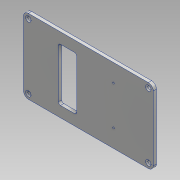
# Autodesk Inventor part: AK-C-C39-Top
Saved by Autodesk Inventor 2016 (Build 200138000, 138)
## iProperties
Created: 2016-04-01
Part Number: AK-C-C39-Top
Material: Aluminum 6061
Document SubType Name: Modeling
Designer: admin
Density: 2.7 g/cm^3
Appearance: Aluminum - Flat
Mass: 59.7394 g
Surface Area: 163.872 cm^2
Volume: 22.1257 cm^3
Author: admin
Autodesk Inventor part; units mm, degrees
ref_plane "YZ Plane" through (0, 0, 0) normal (1, 0, 0) x (0, 1, 0)
ref_plane "XZ Plane" through (0, 0, 0) normal (0, 1, 0) x (-1, 0, 0)
ref_plane "XY Plane" through (0, 0, 0) normal (0, 0, 1) x (1, 0, 0)
derived "AK-C-C39-Main-Board.ipt"
sketch "Sketch1" plane through (0, 0, 0) normal (0, 1, 0) x (-1, 0, 0)
  line L0 (-55, -17.425) -> (-56.5, -17.425)
  line L1 (-56.5, -17.425) -> (-56.5, -16.775)
  line L2 (-58.5, -16.775) -> (-58.5, -17.425)
  line L3 (-58.5, -17.425) -> (-60, -17.425)
  line L4 (-60, -29.925) -> (-60, -17.425)
  line L5 (-60, -16.775) -> (-60, 29.925)
  line L6 (55, -17.425) -> (56.5, -17.425)
  line L7 (58.5, -17.425) -> (60, -17.425)
  line L8 (60, -29.925) -> (60, -17.425)
  line L9 (60, -16.775) -> (60, 29.925)
  arc A0 (-52.8, -29.7756) -> (-53.6536, -29.4221) centre (-53.3, -29.7756) ccw
  arc A1 (-54.9971, -28.0786) -> (-55.3506, -27.225) centre (-55.3506, -27.725) ccw
  line L10 (-54.2538, -30.0223) -> (-53.6536, -29.4221)
  line L11 (-55.5973, -28.6788) -> (-54.9971, -28.0786)
  arc A2 (54.9971, 28.0786) -> (55.3506, 27.225) centre (55.3506, 27.725) ccw
  line L12 (55.5, 29.925) -> (51.9091, 26.3341) construction
  arc A3 (52.8, 29.7756) -> (53.6536, 29.4221) centre (53.3, 29.7756) ccw
  line L13 (55, -16.775) -> (56.5, -16.775)
  line L14 (58.5, -16.775) -> (60, -16.775)
  line L15 (57.8, -3.3607) -> (55, -7.6074)
  line L16 (55, -7.6074) -> (55, -16.775)
  arc A4 (56.5, -18.525) -> (58.5, -18.525) centre (57.5, -19.275) ccw
  line L17 (58.5, -18.525) -> (58.5, -16.775)
  line L18 (56.5, -18.525) -> (56.5, -16.775)
  line L19 (-55.5973, 28.6788) -> (-54.9971, 28.0786)
  line L20 (-54.2538, 30.0223) -> (-53.6536, 29.4221)
  arc A5 (-53.6536, 29.4221) -> (-52.8, 29.7756) centre (-53.3, 29.7756) ccw
  arc A6 (-55.3506, 27.225) -> (-54.9971, 28.0786) centre (-55.3506, 27.725) ccw
  line L21 (-57.8, -3.3607) -> (-55, -7.6074)
  line L22 (-55, -7.6074) -> (-55, -16.775)
  arc A7 (-56.5, -15.025) -> (-58.5, -15.025) centre (-57.5, -14.275) ccw
  line L23 (-58.5, -15.025) -> (-58.5, -16.775)
  line L24 (-56.5, -15.025) -> (-56.5, -16.775)
  line L25 (-55, -16.775) -> (-56.5, -16.775)
  line L26 (-58.5, -16.775) -> (-60, -16.775)
  line L27 (57.5, -16.4962) -> (57.5, -11.7384) construction
  line L28 (-52.8, -31.925) -> (-52.8, -29.7756)
  line L29 (-55.3506, -27.225) -> (-57.5, -27.225)
  line L30 (-57.5, -27.225) -> (-57.5, -25.225)
  line L31 (-57.5, -25.225) -> (-55, -25.225)
  line L32 (-55, -25.225) -> (-55, -17.425)
  line L33 (48.8, -31.925) -> (46.8, -31.925)
  line L34 (46.8, -31.925) -> (46.8, -29.925)
  line L35 (46.8, -29.925) -> (44.8, -29.925)
  line L36 (44.8, -29.925) -> (44.8, -32.325)
  line L37 (-44.8, -32.325) -> (-44.8, -29.925)
  line L38 (-44.8, -29.925) -> (-46.8, -29.925)
  line L39 (-46.8, -29.925) -> (-46.8, -31.925)
  line L40 (-46.8, -31.925) -> (-48.8, -31.925)
  line L41 (-48.8, -31.925) -> (-48.8, -29.925)
  line L42 (-48.8, -29.925) -> (-50.8, -29.925)
  line L43 (-50.8, -29.925) -> (-50.8, -31.925)
  line L44 (-50.8, -31.925) -> (-52.8, -31.925)
  line L45 (55, -17.425) -> (55, -25.225)
  line L46 (55, -25.225) -> (57.5, -25.225)
  line L47 (57.5, -25.225) -> (57.5, -27.225)
  line L48 (57.5, -27.225) -> (55.3506, -27.225)
  line L49 (52.8, -29.7756) -> (52.8, -31.925)
  line L50 (52.8, -31.925) -> (50.8, -31.925)
  line L51 (50.8, -31.925) -> (50.8, -29.925)
  line L52 (50.8, -29.925) -> (48.8, -29.925)
  line L53 (48.8, -29.925) -> (48.8, -31.925)
  line L54 (5, -32.325) -> (5, -29.925)
  line L55 (5, -29.925) -> (3, -29.925)
  line L56 (3, -29.925) -> (3, -31.925)
  line L57 (3, -31.925) -> (1, -31.925)
  line L58 (1, -31.925) -> (1, -29.925)
  line L59 (1, -29.925) -> (-1, -29.925)
  line L60 (-1, -29.925) -> (-1, -31.925)
  line L61 (-1, -31.925) -> (-3, -31.925)
  line L62 (-3, -31.925) -> (-3, -29.925)
  line L63 (-3, -29.925) -> (-5, -29.925)
  line L64 (-5, -29.925) -> (-5, -32.325)
  line L65 (-5, -32.325) -> (-44.8, -32.325)
  line L66 (44.8, -32.325) -> (5, -32.325)
  line L67 (-57.5, -20.9142) -> (-57.5, -16.6435) construction
  arc A8 (60, 29.925) -> (55.5, 34.425) centre (55.5, 29.925) ccw
  arc A9 (-55.5, 34.425) -> (-60, 29.925) centre (-55.5, 29.925) ccw
  arc A10 (-60, -29.925) -> (-55.5, -34.425) centre (-55.5, -29.925) ccw
  line L68 (57.5, 27.225) -> (57.5, 25.225)
  line L69 (57.5, 25.225) -> (55.5, 25.225)
  line L70 (55.5, 25.225) -> (55.5, 23.225)
  line L71 (55.5, 23.225) -> (57.5, 23.225)
  line L72 (57.5, 23.225) -> (57.5, 21.225)
  line L73 (57.5, 21.225) -> (55.5, 21.225)
  line L74 (55.5, 21.225) -> (55.5, 19.225)
  line L75 (55.5, 19.225) -> (57.8, 19.225)
  line L76 (57.8, 19.225) -> (57.8, -3.3607)
  line L77 (3, 31.925) -> (1, 31.925)
  line L78 (1, 31.925) -> (1, 29.925)
  line L79 (1, 29.925) -> (-1, 29.925)
  line L80 (-1, 29.925) -> (-1, 31.925)
  line L81 (-1, 31.925) -> (-3, 31.925)
  line L82 (-3, 31.925) -> (-3, 29.925)
  line L83 (-3, 29.925) -> (-5, 29.925)
  line L84 (-5, 29.925) -> (-5, 32.325)
  line L85 (-5, 32.325) -> (-44.8, 32.325)
  line L86 (-44.8, 32.325) -> (-44.8, 29.925)
  line L87 (-44.8, 29.925) -> (-46.8, 29.925)
  line L88 (-46.8, 29.925) -> (-46.8, 31.925)
  line L89 (-46.8, 31.925) -> (-48.8, 31.925)
  line L90 (-48.8, 31.925) -> (-48.8, 29.925)
  line L91 (-48.8, 29.925) -> (-50.8, 29.925)
  line L92 (-50.8, 29.925) -> (-50.8, 31.925)
  line L93 (-50.8, 31.925) -> (-52.8, 31.925)
  line L94 (-52.8, 31.925) -> (-52.8, 29.7756)
  line L95 (-55.3506, 27.225) -> (-57.5, 27.225)
  line L96 (55.5973, 28.6788) -> (54.9971, 28.0786)
  line L97 (54.2538, 30.0223) -> (53.6536, 29.4221)
  line L98 (57.5, 27.225) -> (55.3506, 27.225)
  line L99 (52.8, 29.7756) -> (52.8, 31.925)
  line L100 (52.8, 31.925) -> (50.8, 31.925)
  line L101 (50.8, 31.925) -> (50.8, 29.925)
  line L102 (50.8, 29.925) -> (48.8, 29.925)
  line L103 (48.8, 29.925) -> (48.8, 31.925)
  line L104 (48.8, 31.925) -> (46.8, 31.925)
  line L105 (46.8, 31.925) -> (46.8, 29.925)
  line L106 (46.8, 29.925) -> (44.8, 29.925)
  line L107 (44.8, 29.925) -> (44.8, 32.325)
  line L108 (44.8, 32.325) -> (5, 32.325)
  line L109 (5, 32.325) -> (5, 29.925)
  line L110 (5, 29.925) -> (3, 29.925)
  line L111 (3, 29.925) -> (3, 31.925)
  line L112 (-57.5, 27.225) -> (-57.5, 25.225)
  line L113 (-57.5, 25.225) -> (-55.5, 25.225)
  line L114 (-55.5, 25.225) -> (-55.5, 23.225)
  line L115 (-55.5, 23.225) -> (-57.5, 23.225)
  line L116 (-57.5, 23.225) -> (-57.5, 21.225)
  line L117 (-57.5, 21.225) -> (-55.5, 21.225)
  line L118 (-55.5, 21.225) -> (-55.5, 19.225)
  line L119 (-55.5, 19.225) -> (-57.8, 19.225)
  line L120 (-57.8, 19.225) -> (-57.8, -3.3607)
  line L121 (55.5, -34.425) -> (-55.5, -34.425)
  line L122 (9.5866, 0) -> (-6.7847, 0) construction
  line L123 (0, -6.6233) -> (0, 6.4737) construction
  arc A11 (55.5, -34.425) -> (60, -29.925) centre (55.5, -29.925) ccw
  arc A12 (55.3506, -27.225) -> (54.9971, -28.0786) centre (55.3506, -27.725) ccw
  arc A13 (53.6536, -29.4221) -> (52.8, -29.7756) centre (53.3, -29.7756) ccw
  line L124 (54.9971, -28.0786) -> (55.5973, -28.6788)
  line L125 (53.6536, -29.4221) -> (54.2538, -30.0223)
  arc A14 (55.5973, 28.6788) -> (54.2538, 30.0223) centre (55.5, 29.925) ccw
  arc A15 (-54.2538, 30.0223) -> (-55.5973, 28.6788) centre (-55.5, 29.925) ccw
  arc A16 (54.2538, -30.0223) -> (55.5973, -28.6788) centre (55.5, -29.925) ccw
  arc A17 (-55.5973, -28.6788) -> (-54.2538, -30.0223) centre (-55.5, -29.925) ccw
  line L126 (55.5, 34.425) -> (-55.5, 34.425)
  point P0 (0, 0)
sketch "Sketch2" plane through (0, 0, 0) normal (0, 1, 0) x (-1, 0, 0)
  line L0 (51.25, -29) -> (44.125, -29)
  line L1 (43.25, -29.875) -> (43.25, -31)
  line L2 (43.25, -31) -> (6.5, -31)
  line L3 (6.5, -31) -> (6.5, -29.875)
  line L4 (5.625, -29) -> (-5.625, -29)
  line L5 (-6.5, -29.875) -> (-6.5, -31)
  line L6 (-6.5, -31) -> (-43.25, -31)
  line L7 (-43.25, -31) -> (-43.25, -29.875)
  line L8 (-44.125, -29) -> (-51.25, -29)
  line L9 (-51.25, -29) -> (-53.75, -26.5)
  line L10 (-53.75, -26.5) -> (-53.75, 26.5)
  line L11 (-53.75, 26.5) -> (-51.25, 29)
  line L12 (-51.25, 29) -> (-44.125, 29)
  line L13 (-43.25, 29.875) -> (-43.25, 31)
  line L14 (-43.25, 31) -> (-6.5, 31)
  line L15 (-6.5, 31) -> (-6.5, 29.875)
  line L16 (-5.625, 29) -> (5.625, 29)
  line L17 (6.5, 29.875) -> (6.5, 31)
  line L18 (43.25, 31) -> (43.25, 29.875)
  line L19 (43.25, 31) -> (6.5, 31)
  line L20 (44.125, 29) -> (51.25, 29)
  line L21 (51.25, 29) -> (53.75, 26.5)
  line L22 (53.75, 26.5) -> (53.75, -26.5)
  line L23 (53.75, -26.5) -> (51.25, -29)
  line L24 (44.8, -32.325) -> (5, -32.325)
  line L25 (5, -32.325) -> (5, -29.925)
  line L26 (5, -29.925) -> (3, -29.925)
  line L27 (44.8, -29.925) -> (44.8, -32.325)
  line L28 (46.8, -29.925) -> (44.8, -29.925)
  line L29 (52.8, -29.7756) -> (52.8, -31.925)
  arc A0 (53.6536, -29.4221) -> (52.8, -29.7756) centre (53.3, -29.7756) ccw
  arc A1 (55.3506, -27.225) -> (54.9971, -28.0786) centre (55.3506, -27.725) ccw
  line L30 (55, -17.425) -> (55, -25.225)
  line L31 (0, -6.6233) -> (0, 6.4737) construction
  line L32 (9.5866, 0) -> (-6.7847, 0) construction
  line L33 (57.8, 19.225) -> (57.8, -3.3607)
  line L34 (57.8, -3.3607) -> (55, -7.6074)
  line L35 (55.5, 19.225) -> (57.8, 19.225)
  line L36 (55.5, 29.925) -> (51.9091, 26.3341) construction
  line L37 (25.75, -24.5) -> (12.75, -24.5)
  line L38 (12.75, 24.5) -> (25.75, 24.5)
  line L39 (3.3524, -20) -> (-16.6476, -20)
  line L40 (-16.6476, -20) -> (-16.6476, 20)
  line L41 (-16.6476, 20) -> (3.3524, 20)
  line L42 (3.3524, 20) -> (3.3524, -20)
  line L43 (-23.9878, -15) -> (-31.9878, -15) construction
  line L44 (-31.9878, -15) -> (-31.9878, -7) construction
  line L45 (-31.9878, -7) -> (-23.9878, -7) construction
  line L46 (-23.9878, -7) -> (-23.9878, -15) construction
  line L47 (-34.9878, -15) -> (-42.9878, -15) construction
  line L48 (-42.9878, -15) -> (-42.9878, -7) construction
  line L49 (-42.9878, -7) -> (-34.9878, -7) construction
  line L50 (-34.9878, -7) -> (-34.9878, -15) construction
  line L51 (-23.9878, -4) -> (-31.9878, -4) construction
  line L52 (-31.9878, -4) -> (-31.9878, 4) construction
  line L53 (-31.9878, 4) -> (-23.9878, 4) construction
  line L54 (-23.9878, 4) -> (-23.9878, -4) construction
  line L55 (-34.9878, -4) -> (-42.9878, -4) construction
  line L56 (-42.9878, -4) -> (-42.9878, 4) construction
  line L57 (-42.9878, 4) -> (-34.9878, 4) construction
  line L58 (-34.9878, 4) -> (-34.9878, -4) construction
  line L59 (-23.9878, 7) -> (-31.9878, 7) construction
  line L60 (-31.9878, 7) -> (-31.9878, 15) construction
  line L61 (-31.9878, 15) -> (-23.9878, 15) construction
  line L62 (-23.9878, 15) -> (-23.9878, 7) construction
  line L63 (-34.9878, 7) -> (-42.9878, 7) construction
  line L64 (-42.9878, 7) -> (-42.9878, 15) construction
  line L65 (-42.9878, 15) -> (-34.9878, 15) construction
  line L66 (-34.9878, 15) -> (-34.9878, 7) construction
  line L67 (25.75, -22.5) -> (12.75, -22.5) construction
  line L68 (12.75, -22.5) -> (12.75, -9.5) construction
  line L69 (12.75, -9.5) -> (25.75, -9.5) construction
  line L70 (25.75, -9.5) -> (25.75, -22.5) construction
  line L71 (25.75, -6.5) -> (12.75, -6.5) construction
  line L72 (12.75, -6.5) -> (12.75, 6.5) construction
  line L73 (12.75, 6.5) -> (25.75, 6.5) construction
  line L74 (25.75, 6.5) -> (25.75, -6.5) construction
  line L75 (25.75, 9.5) -> (12.75, 9.5) construction
  line L76 (12.75, 9.5) -> (12.75, 22.5) construction
  line L77 (12.75, 22.5) -> (25.75, 22.5) construction
  line L78 (25.75, 22.5) -> (25.75, 9.5) construction
  line L79 (31.9633, -16) -> (17.7262, -16) construction
  line L80 (31.9633, 16) -> (18.8213, 16) construction
  line L81 (19.25, -23.7063) -> (19.25, 24.6931) construction
  arc A2 (10.75, -22.5) -> (12.75, -24.5) centre (12.75, -22.5) ccw
  arc A3 (25.75, -24.5) -> (27.75, -22.5) centre (25.75, -22.5) ccw
  arc A4 (12.75, 24.5) -> (10.75, 22.5) centre (12.75, 22.5) ccw
  arc A5 (27.75, 22.5) -> (25.75, 24.5) centre (25.75, 22.5) ccw
  line L82 (55, -25.225) -> (-54.9956, -25.225) construction
  line L83 (55.5, 25.225) -> (55.5, 23.225)
  line L84 (57.5, 25.225) -> (55.5, 25.225)
  line L85 (-57.5, 25.225) -> (-55.5, 25.225)
  line L86 (-55.5, 25.225) -> (-55.5, 23.225)
  line L87 (-57.5, -25.225) -> (-55, -25.225)
  line L88 (-55, -25.225) -> (-55, -17.425)
  line L89 (55, -25.225) -> (57.5, -25.225)
  line L90 (55.5, 25.225) -> (-55.5, 25.225) construction
  line L91 (48.25, -2.5) -> (48.25, 2.5)
  line L92 (50, -2.5) -> (50, 2.5)
  line L93 (50, -4) -> (48.25, -4)
  line L94 (50, 4) -> (48.25, 4)
  arc A6 (50, -4) -> (50, -2.5) centre (50, -3.25) ccw
  arc A7 (48.25, -2.5) -> (48.25, -4) centre (48.25, -3.25) ccw
  arc A8 (50, 2.5) -> (50, 4) centre (50, 3.25) ccw
  arc A9 (48.25, 4) -> (48.25, 2.5) centre (48.25, 3.25) ccw
  line L95 (-37.75, -2.5) -> (-37.75, 2.5)
  line L96 (-39.5, 4) -> (-37.75, 4)
  line L97 (-39.5, 2.5) -> (-39.5, -2.5)
  line L98 (-39.5, -4) -> (-37.75, -4)
  arc A10 (-37.75, -4) -> (-37.75, -2.5) centre (-37.75, -3.25) ccw
  arc A11 (-39.5, -2.5) -> (-39.5, -4) centre (-39.5, -3.25) ccw
  arc A12 (-37.75, 2.5) -> (-37.75, 4) centre (-37.75, 3.25) ccw
  arc A13 (-39.5, 4) -> (-39.5, 2.5) centre (-39.5, 3.25) ccw
  line L99 (48.75, -27) -> (40.5, -27)
  line L100 (38.75, -27) -> (38.75, -25.25)
  line L101 (40.5, -25.25) -> (48.75, -25.25)
  line L102 (1.75, -27) -> (-8.25, -27)
  line L103 (-8.25, -25.25) -> (1.75, -25.25)
  line L104 (-40, -27) -> (-48.25, -27)
  line L105 (-48.25, -25.25) -> (-40, -25.25)
  line L106 (-48.25, 25.25) -> (-40, 25.25)
  line L107 (-40, 27) -> (-48.25, 27)
  line L108 (1.75, 25.25) -> (-8.25, 25.25)
  line L109 (-8.25, 27) -> (1.75, 27)
  line L110 (48.75, 25.25) -> (40.25, 25.25)
  line L111 (38.75, 25.25) -> (38.75, 27)
  line L112 (40.25, 27) -> (48.75, 27)
  arc A14 (38.75, -27) -> (40.5, -27) centre (39.625, -27) ccw
  arc A15 (40.5, -25.25) -> (38.75, -25.25) centre (39.625, -25.25) ccw
  arc A16 (38.75, 25.25) -> (40.25, 25.25) centre (39.5, 25.25) ccw
  arc A17 (40.25, 27) -> (38.75, 27) centre (39.5, 27) ccw
  line L113 (27.75, 22.5) -> (27.75, -22.5)
  line L114 (-34.9878, 7) -> (-42.9878, 15) construction
  line L115 (-31.9878, 7) -> (-23.9878, 15) construction
  line L116 (-31.9878, -7) -> (-23.9878, -15) construction
  line L117 (-34.9878, -7) -> (-42.9878, -15) construction
  arc A18 (3.3524, 19) -> (2.3524, 20) centre (2.3524, 19) ccw
  arc A19 (-15.6476, 20) -> (-16.6476, 19) centre (-15.6476, 19) ccw
  arc A20 (2.3524, -20) -> (3.3524, -19) centre (2.3524, -19) ccw
  arc A21 (-16.6476, -19) -> (-15.6476, -20) centre (-15.6476, -19) ccw
  line L118 (10.75, 7.999) -> (10.75, 8)
  line L119 (10.75, -22.5) -> (10.75, 22.5)
  arc A22 (48.75, 25.25) -> (48.75, 27) centre (48.75, 26.125) ccw
  arc A23 (-8.25, 27) -> (-8.25, 25.25) centre (-8.25, 26.125) ccw
  arc A24 (-48.25, 27) -> (-48.25, 25.25) centre (-48.25, 26.125) ccw
  arc A25 (48.75, -27) -> (48.75, -25.25) centre (48.75, -26.125) ccw
  arc A26 (-8.25, -25.25) -> (-8.25, -27) centre (-8.25, -26.125) ccw
  arc A27 (-48.25, -25.25) -> (-48.25, -27) centre (-48.25, -26.125) ccw
  line L120 (31, 25) -> (29.25, 25)
  line L121 (31, 23.5) -> (31, 20)
  line L122 (29.25, 20) -> (29.25, 23.5)
  arc A28 (31, 23.5) -> (31, 25) centre (31, 24.25) ccw
  arc A29 (29.25, 25) -> (29.25, 23.5) centre (29.25, 24.25) ccw
  arc A30 (29.25, 20) -> (31, 20) centre (30.125, 20) ccw
  line L123 (29.25, -20) -> (29.25, -23.25)
  line L124 (29.25, -25) -> (31, -25)
  line L125 (31, -23.25) -> (31, -20)
  arc A31 (31, -25) -> (31, -23.25) centre (31, -24.125) ccw
  arc A32 (29.25, -23.25) -> (29.25, -25) centre (29.25, -24.125) ccw
  arc A33 (31, -20) -> (29.25, -20) centre (30.125, -20) ccw
  line L126 (9.25, 25) -> (7.5, 25)
  line L127 (7.5, 23.5) -> (7.5, 20)
  line L128 (9.25, 20) -> (9.25, 23.5)
  line L129 (7.5, -20) -> (7.5, -23.25)
  line L130 (7.5, -25) -> (9.25, -25)
  line L131 (9.25, -23.25) -> (9.25, -20)
  arc A34 (9.25, -20) -> (7.5, -20) centre (8.375, -20) ccw
  arc A35 (9.25, -25) -> (9.25, -23.25) centre (9.25, -24.125) ccw
  arc A36 (7.5, -23.25) -> (7.5, -25) centre (7.5, -24.125) ccw
  arc A37 (7.5, 20) -> (9.25, 20) centre (8.375, 20) ccw
  arc A38 (9.25, 23.5) -> (9.25, 25) centre (9.25, 24.25) ccw
  arc A39 (7.5, 25) -> (7.5, 23.5) centre (7.5, 24.25) ccw
  line L132 (29.25, 4) -> (29.25, -4)
  line L133 (31, -4) -> (31, 4)
  line L134 (7.5, 4) -> (7.5, -4)
  line L135 (9.25, -4) -> (9.25, 4)
  arc A40 (31, 4) -> (29.25, 4) centre (30.125, 4) ccw
  arc A41 (29.25, -4) -> (31, -4) centre (30.125, -4) ccw
  arc A42 (9.25, 4) -> (7.5, 4) centre (8.375, 4) ccw
  arc A43 (7.5, -4) -> (9.25, -4) centre (8.375, -4) ccw
  line L136 (-14.75, 30.3253) -> (-31.75, 30.3253) construction
  line L137 (-31.75, 30.3253) -> (-31.75, 22.4164) construction
  line L138 (-31.75, 22.4164) -> (-14.75, 22.4164) construction
  line L139 (-14.75, 22.4164) -> (-14.75, 30.3253) construction
  line L140 (-23.25, 29.9722) -> (-23.25, 20.9797) construction
  arc A44 (6.5, -29.875) -> (5.625, -29) centre (5.625, -29.875) ccw
  arc A45 (-5.625, -29) -> (-6.5, -29.875) centre (-5.625, -29.875) ccw
  arc A46 (-43.25, -29.875) -> (-44.125, -29) centre (-44.125, -29.875) ccw
  arc A47 (-44.125, 29) -> (-43.25, 29.875) centre (-44.125, 29.875) ccw
  arc A48 (-6.5, 29.875) -> (-5.625, 29) centre (-5.625, 29.875) ccw
  arc A49 (5.625, 29) -> (6.5, 29.875) centre (5.625, 29.875) ccw
  arc A50 (43.25, 29.875) -> (44.125, 29) centre (44.125, 29.875) ccw
  arc A51 (44.125, -29) -> (43.25, -29.875) centre (44.125, -29.875) ccw
  line L141 (57.5, 27.225) -> (57.5, 25.225)
  line L142 (-57.5, 27.225) -> (-57.5, 25.225)
  arc A52 (1.75, 25.25) -> (1.75, 27) centre (1.75, 26.125) ccw
  arc A53 (1.75, -27) -> (1.75, -25.25) centre (1.75, -26.125) ccw
  arc A54 (-38.25, 27) -> (-40, 27) centre (-39.125, 27) ccw
  arc A55 (-40, 25.25) -> (-38.25, 25.25) centre (-39.125, 25.25) ccw
  line L143 (-38.25, 27) -> (-38.25, 25.25)
  arc A56 (-38.25, -25.25) -> (-40, -25.25) centre (-39.125, -25.25) ccw
  arc A57 (-40, -27) -> (-38.25, -27) centre (-39.125, -27) ccw
  line L144 (-38.25, -25.25) -> (-38.25, -27)
  line L145 (-60, -16.775) -> (-60, 29.925)
  point P0 (53.75, -25.225)
  point P1 (25.75, -16)
  point P2 (25.75, 16)
  point P3 (19.25, -22.5)
  point P4 (19.25, -24.5)
  point P5 (27.75, 0)
  point P6 (10.75, 0)
  point P7 (-23.25, 30.3253)
  point P8 (-23.25, 18)
  point P9 (-23.25, -18)
  point P10 (-53.75, -25.225)
  dimension "d33" = 2
  measures "d33" diameter of A19
sketch "Sketch3" plane through (0, 0, 0) normal (0, 1, 0) x (-1, 0, 0)
  line L0 (55.5, -34.425) -> (-55.5, -34.425) projected
  arc A0 (55.5, -34.425) -> (60, -29.925) centre (55.5, -29.925) ccw projected
  line L1 (60, -29.925) -> (60, -17.425) projected
  line L2 (60, -16.775) -> (60, 29.925) projected
  arc A1 (60, 29.925) -> (55.5, 34.425) centre (55.5, 29.925) ccw projected
  line L3 (55.5, 34.425) -> (-55.5, 34.425) projected
  arc A2 (-55.5, 34.425) -> (-60, 29.925) centre (-55.5, 29.925) ccw projected
  line L4 (-60, -16.775) -> (-60, 29.925) projected
  line L5 (-60, -29.925) -> (-60, -17.425) projected
  arc A3 (-60, -29.925) -> (-55.5, -34.425) centre (-55.5, -29.925) ccw projected
  line L6 (60, -17.425) -> (60, -16.775)
  line L7 (-60, -17.425) -> (-60, -16.775)
  point P0 (0, 0)
  constraints: 4 end point, 1 parallel, 1 vertical
extrude "Extrusion1" add sketch "Sketch3" along normal blind 3
hole "Hole1" at (-55.5, 0, 29.925) at (55.5, 0, 29.925) at (-55.5, 0, -29.925) at (55.5, 0, -29.925) direction (0, 1, 0) diameter 3 end through all countersink diameter 5 countersink angle 90
extrude "Extrusion3" [suppressed]
sketch "Sketch5" plane through (0, 0, 0) normal (0, -1, 0) x (1, 0, 0)
  line L0 (23.9878, 15) -> (23.9878, 7) projected
  line L1 (31.9878, 15) -> (23.9878, 15) projected
  line L2 (31.9878, 7) -> (31.9878, 15) projected
  line L3 (23.9878, 7) -> (31.9878, 7) projected
  line L4 (31.9878, 4) -> (23.9878, 4) projected
  line L5 (23.9878, 4) -> (23.9878, -4) projected
  line L6 (23.9878, -4) -> (31.9878, -4) projected
  line L7 (31.9878, -4) -> (31.9878, 4) projected
  line L8 (31.9878, -7) -> (23.9878, -7) projected
  line L9 (23.9878, -7) -> (23.9878, -15) projected
  line L10 (23.9878, -15) -> (31.9878, -15) projected
  line L11 (31.9878, -15) -> (31.9878, -7) projected
  line L12 (34.9878, -7) -> (34.9878, -15) projected
  line L13 (34.9878, -15) -> (42.9878, -15) projected
  line L14 (42.9878, -15) -> (42.9878, -7) projected
  line L15 (42.9878, -7) -> (34.9878, -7) projected
  line L16 (34.9878, -4) -> (42.9878, -4) projected
  line L17 (34.9878, 4) -> (34.9878, -4) projected
  line L18 (42.9878, 4) -> (34.9878, 4) projected
  line L19 (42.9878, -4) -> (42.9878, 4) projected
  line L20 (42.9878, 7) -> (42.9878, 15) projected
  line L21 (42.9878, 15) -> (34.9878, 15) projected
  line L22 (34.9878, 15) -> (34.9878, 7) projected
  line L23 (34.9878, 7) -> (42.9878, 7) projected
  arc A0 (23.9878, -14) -> (24.9878, -15) centre (24.9878, -14) ccw
  arc A1 (24.9878, -7) -> (23.9878, -8) centre (24.9878, -8) ccw
  arc A2 (30.9878, -15) -> (31.9878, -14) centre (30.9878, -14) ccw
  arc A3 (31.9878, -8) -> (30.9878, -7) centre (30.9878, -8) ccw
  arc A4 (34.9878, -14) -> (35.9878, -15) centre (35.9878, -14) ccw
  arc A5 (35.9878, -7) -> (34.9878, -8) centre (35.9878, -8) ccw
  arc A6 (41.9878, -15) -> (42.9878, -14) centre (41.9878, -14) ccw
  arc A7 (42.9878, -8) -> (41.9878, -7) centre (41.9878, -8) ccw
  arc A8 (34.9878, -3) -> (35.9878, -4) centre (35.9878, -3) ccw
  arc A9 (35.9878, 4) -> (34.9878, 3) centre (35.9878, 3) ccw
  arc A10 (41.9878, -4) -> (42.9878, -3) centre (41.9878, -3) ccw
  arc A11 (42.9878, 3) -> (41.9878, 4) centre (41.9878, 3) ccw
  arc A12 (23.9878, -3) -> (24.9878, -4) centre (24.9878, -3) ccw
  arc A13 (24.9878, 4) -> (23.9878, 3) centre (24.9878, 3) ccw
  arc A14 (30.9878, -4) -> (31.9878, -3) centre (30.9878, -3) ccw
  arc A15 (31.9878, 3) -> (30.9878, 4) centre (30.9878, 3) ccw
  arc A16 (23.9878, 8) -> (24.9878, 7) centre (24.9878, 8) ccw
  arc A17 (24.9878, 15) -> (23.9878, 14) centre (24.9878, 14) ccw
  arc A18 (30.9878, 7) -> (31.9878, 8) centre (30.9878, 8) ccw
  arc A19 (31.9878, 14) -> (30.9878, 15) centre (30.9878, 14) ccw
  arc A20 (34.9878, 8) -> (35.9878, 7) centre (35.9878, 8) ccw
  arc A21 (35.9878, 15) -> (34.9878, 14) centre (35.9878, 14) ccw
  arc A22 (41.9878, 7) -> (42.9878, 8) centre (41.9878, 8) ccw
  arc A23 (42.9878, 14) -> (41.9878, 15) centre (41.9878, 14) ccw
  point P0 (0, 0)
  dimension "d16" = 2
  constraints: 48 point on circle, 48 point on line, 48 tangent, 24 centre point, 23 equal radius
  measures "d16" diameter of A0
extrude "Extrusion5" [suppressed]
sketch "Sketch6" plane through (0, 0, 0) normal (0, -1, 0) x (1, 0, 0)
  point P0 (0, 0)
  point P1 (23.25, 18)
  point P2 (23.25, -18)
hole "Hole3" at (23.25, 0, 18) at (23.25, 0, -18) direction (0, 1, 0) diameter 1.567 depth 35.169 tip angle 118 thread size "M2x0.4" class "6H" standard "ANSI Metric M Profile"
extrude "Extrusion6" cut sketch "Sketch2" along normal blind 10 contours L37 A2 L119 A4 L38 A5 L113 A3
body "Solid1"
